Autodesk Inventor part; units mm, degrees
(part 13 of 13)
sketch "Sketch2" plane through (0, 0, 0) normal (0, 1, 0) x (-1, 0, 0)
  line L0 (-22.8128, 17.9045) -> (22.9025, 17.9045)
  line L1 (-26.8635, 14.0674) -> (-26.8635, -13.9573)
  line L2 (-23.0317, -17.859) -> (22.9423, -17.859)
  line L3 (26.7728, 14.0731) -> (26.7728, -14.1827)
  circle A0 centre (-24.1817, 15.2166) radius 1.1494
  circle A1 centre (-24.1817, -15.1773) radius 1.1495
  circle A2 centre (24.091, -15.1773) radius 1.1495
  circle A3 centre (24.091, 15.2166) radius 1.1494
  arc A4 (-22.8128, 17.9045) -> (-26.8635, 14.0674) centre (-22.8128, 13.8478) ccw
  arc A5 (26.7728, 14.0731) -> (22.9025, 17.9045) centre (22.9025, 14.034) ccw
  arc A6 (-26.8635, -13.9573) -> (-23.0317, -17.859) centre (-22.9612, -13.9573) ccw
  arc A7 (22.9423, -17.859) -> (26.7728, -14.1827) centre (23.0934, -14.1827) ccw
  line L4 (-26.8635, 0.055) -> (26.7728, -0.0548) construction
  line L5 (0.0448, 17.9045) -> (-0.0447, -17.859) construction
  line L6 (22.9025, 18.4045) -> (-22.8128, 18.4045)
  arc A8 (-22.8128, 18.4045) -> (-27.3635, 14.0805) centre (-22.8128, 13.8478) ccw
  line L7 (-27.3635, 14.0805) -> (-27.3635, -13.9573)
  arc A9 (-27.3635, -13.9573) -> (-23.0361, -18.359) centre (-22.9612, -13.9573) ccw
  line L8 (-23.0361, -18.359) -> (22.9323, -18.359)
  arc A10 (22.9323, -18.359) -> (27.2728, -14.1827) centre (23.0934, -14.1827) ccw
  line L9 (27.2728, -14.1827) -> (27.2728, 14.0756)
  arc A11 (27.2728, 14.0756) -> (22.9025, 18.4045) centre (22.9025, 14.034) ccw
  line L10 (-22.8128, 20.4045) -> (22.9025, 20.4045)
  arc A12 (29.2728, 14.0842) -> (22.9025, 20.4045) centre (22.9025, 14.034) ccw
  line L11 (29.2728, 14.0842) -> (29.2728, -14.1827)
  arc A13 (22.8975, -20.359) -> (29.2728, -14.1827) centre (23.0934, -14.1827) ccw
  line L12 (22.8975, -20.359) -> (-23.0515, -20.359)
  arc A14 (-29.3635, -13.9573) -> (-23.0515, -20.359) centre (-22.9612, -13.9573) ccw
  line L13 (-29.3635, -13.9573) -> (-29.3635, 14.127)
  arc A15 (-22.8128, 20.4045) -> (-29.3635, 14.127) centre (-22.8128, 13.8478) ccw
  circle A16 centre (-24.1817, 15.2166) radius 1.7494
  arc A17 (-27.3635, 13.2331) -> (-22.2079, 18.4045) centre (-24.1817, 15.2166) ccw
  circle A18 centre (24.091, 15.2166) radius 1.7494
  arc A19 (22.1171, 18.4045) -> (27.2728, 13.2331) centre (24.091, 15.2166) ccw
  circle A20 centre (24.091, -15.1773) radius 1.7495
  arc A21 (27.2728, -13.1938) -> (22.1073, -18.359) centre (24.091, -15.1773) ccw
  circle A22 centre (-24.1817, -15.1773) radius 1.7495
  arc A23 (-22.1981, -18.359) -> (-27.3635, -13.1937) centre (-24.1817, -15.1773) ccw
  arc A24 (-22.2079, 18.4045) -> (-27.3635, 13.2331) centre (-24.1817, 15.2166) ccw
  arc A25 (27.2728, 13.2331) -> (22.1171, 18.4045) centre (24.091, 15.2166) ccw
  arc A26 (22.1073, -18.359) -> (27.2728, -13.1938) centre (24.091, -15.1773) ccw
  arc A27 (-27.3635, -13.1937) -> (-22.1981, -18.359) centre (-24.1817, -15.1773) ccw
  line L14 (15.9339, -12.0278) -> (33.4909, -12.0278)
  line L15 (15.9339, -1.0278) -> (33.4909, -1.0278)
  point P0 (0, 0)
  point P1 (0, 0)
  dimension "d2" = 0.5
  dimension "d3" = 2
  dimension "d4" = 0.6
  dimension "d5" = 2
  dimension "d6" = 0.6
  dimension "d7" = 2
  dimension "d8" = 0.6
  dimension "d9" = 2
  dimension "d10" = 0.6
  dimension "d11" = 2
  dimension "d22" = 2
  dimension "d23" = 11
  constraints: 40 point on circle, 32 end point, 28 centre point, 10 point on line, 8 coincident, 4 midpoint, 4 tangent, 2 horizontal, 2 vertical, 1 parallel, 1 perpendicular, 22 other
  measures "d2" distance between parallel lines of L0 L6
  measures "d3" distance between parallel lines of L6 L10
  measures "d4" radial gap between concentric circles of A0 A16
  measures "d5" radial gap between concentric circles of A16 A17
  measures "d6" radial gap between concentric circles of A3 A18
  measures "d7" radial gap between concentric circles of A18 A19
  measures "d8" radial gap between concentric circles of A2 A20
  measures "d9" radial gap between concentric circles of A20 A21
  measures "d10" radial gap between concentric circles of A1 A22
  measures "d11" radial gap between concentric circles of A22 A23
  measures "d22" distance edge to line of A2 L14
  measures "d23" distance between parallel lines of L14 L15
extrude "Extrusion1" add sketch "Sketch2" along normal blind 1.5 contours A4 L1 A17 L7 A8 L6 L0 | L0 A17 L1 A4 | A17 L6 A19 L0 | L0 A19 L3 L14 A21 L2 A23 L1 A17 | A19 L6 A11 L9 L3 A5 L0 | L0 A5 L3 A19 | L1 A23 L7 A17 | A24 L7 A27 L8 A26 L9 L14 L11 A13 L12 A14 L13 A15 L10 A12 L15 A25 L6 | L6 A8 L7 A24 | A25 L9 A11 L6 | A19 L9 L15 L3 | A23 L2 A6 L1 | L1 A6 L2 A23 L8 A9 L7 | L15 L9 L14 L3 | L2 A21 L8 A23 | L7 A9 L8 A27 | L15 L11 L14 L9 | L14 L9 A21 L3 | L3 A21 L14 | A21 L14 L3 A7 L2 | L2 A7 L3 A21 L9 A10 L8 | L14 A21 | L8 A10 L9 A26 | A0 | A1 | A2 | A3 | A16 | A18 | A20 | A22
extrude "Extrusion2" cut sketch "Sketch2" along normal blind 1.5 contours A0 | A1 | A2 | A3 | A16 | A18 | A20 | A22
extrude "Extrusion3" add sketch "Sketch2" along normal blind 3 contours A4 L1 A17 L7 A8 L6 L0 | L0 A17 L1 A4 | A19 L6 A11 L9 L3 A5 L0 | L0 A5 L3 A19 | L6 A8 L7 A24 | A25 L9 A11 L6 | A23 L2 A6 L1 | L1 A6 L2 A23 L8 A9 L7 | L7 A9 L8 A27 | A21 L14 L3 A7 L2 | L2 A7 L3 A21 L9 A10 L8 | L14 A21 | L8 A10 L9 A26
extrude "Extrusion4" add sketch "Sketch2" along normal blind 5 contours A24 L7 A27 L8 A26 L9 L14 L11 A13 L12 A14 L13 A15 L10 A12 L15 A25 L6 | L6 A8 L7 A24 | A25 L9 A11 L6 | L7 A9 L8 A27 | L15 L11 L14 L9 | L8 A10 L9 A26
ref_plane "Work Plane1" through (0, 1.5, 0) normal (0, 1, 0) x (-1, 0, 0)
sketch "Sketch3" plane through (0, 1.5, 0) normal (0, 1, 0) x (-1, 0, 0)
  line L0 (30.9565, -1.0278) -> (23.8177, -1.0278)
  line L1 (23.8177, -1.0278) -> (23.8177, -12.0278)
  line L2 (23.8177, -12.0278) -> (30.9565, -12.0278)
  line L3 (30.9565, -12.0278) -> (30.9565, -1.0278)
  line L4 (15.9339, -1.0278) -> (33.4909, -1.0278) projected
  line L5 (15.9339, -12.0278) -> (33.4909, -12.0278) projected
  point P0 (0, 0)
  constraints: 8 end point, 2 collinear, 2 parallel, 1 horizontal, 1 perpendicular
extrude "Extrusion5" cut sketch "Sketch3" along normal blind 5
fillet "Fillet1" radius 2 2 edges at (-28.2728, 5, -1.0278) (-28.2728, 5, -12.0278)
sketch "Sketch4" plane through (0, 0, 0) normal (0, -1, 0) x (1, 0, 0)
  line L0 (-22.306, -6.6429) -> (0.6738, -6.6429) construction
  line L1 (0.6738, -6.6429) -> (0.6738, -10.3811) construction
  line L2 (0.6738, -10.3811) -> (-22.306, -10.3811) construction
  line L3 (-22.306, -10.3811) -> (-22.306, -6.6429) construction
  line L4 (-21.9029, 7.8543) -> (-0.5824, 7.8543) construction
  line L5 (-0.5824, 7.8543) -> (-0.5824, 4.3457) construction
  line L6 (-0.5824, 4.3457) -> (-21.9029, 4.3457) construction
  line L7 (-21.9029, 4.3457) -> (-21.9029, 7.8543) construction
  line L8 (-11.3886, -2.1457) -> (-14.0499, -2.1457)
  line L9 (-14.0499, -2.1457) -> (-14.7437, -0.1294)
  line L10 (-14.7437, -0.1294) -> (-18.4417, -0.1294)
  line L11 (-18.4417, -0.1294) -> (-19.1356, -2.1457)
  line L12 (-19.1356, -2.1457) -> (-21.7396, -2.1457)
  line L13 (-21.7396, -2.1457) -> (-18.0499, 7.8543)
  line L14 (-18.0499, 7.8543) -> (-15.0784, 7.8543)
  line L15 (-15.0784, 7.8543) -> (-11.3886, -2.1457)
  line L16 (-15.3641, 1.7073) -> (-16.5968, 5.2828)
  line L17 (-16.5968, 5.2828) -> (-17.8213, 1.7073)
  line L18 (-17.8213, 1.7073) -> (-15.3641, 1.7073)
  spline S0 degree 2 poles (-1.6907, 4.6951) (-1.6907, 4.0257) (-2.1641, 2.7441) (-2.5968, 2.3032) knots 0 0 0 1 2 2 2
  spline S1 degree 2 poles (-2.5968, 2.3032) (-3.1927, 1.7155) (-4.6703, 1.1114) (-5.7641, 1.1114) knots 0 0 0 1 2 2 2
  line L19 (-5.7641, 1.1114) -> (-7.3723, 1.1114)
  line L20 (-7.3723, 1.1114) -> (-7.3723, -2.1457)
  line L21 (-7.3723, -2.1457) -> (-9.9519, -2.1457)
  line L22 (-9.9519, -2.1457) -> (-9.9519, 7.8543)
  line L23 (-9.9519, 7.8543) -> (-5.707, 7.8543)
  spline S2 degree 2 poles (-5.707, 7.8543) (-4.7519, 7.8543) (-3.4376, 7.5277) (-2.9315, 7.193) knots 0 0 0 1 2 2 2
  spline S3 degree 2 poles (-2.9315, 7.193) (-2.3274, 6.8012) (-1.6907, 5.5604) (-1.6907, 4.6951) knots 0 0 0 1 2 2 2
  spline S4 degree 2 poles (-4.3601, 4.6379) (-4.3601, 5.0624) (-4.8172, 5.6665) (-5.1192, 5.789) knots 0 0 0 1 2 2 2
  spline S5 degree 2 poles (-5.1192, 5.789) (-5.5192, 5.9522) (-6.2866, 5.9849) (-6.9315, 5.9849) knots 0 0 0 1 2 2 2
  line L24 (-6.9315, 5.9849) -> (-7.3723, 5.9849)
  line L25 (-7.3723, 5.9849) -> (-7.3723, 2.9971)
  line L26 (-7.3723, 2.9971) -> (-6.6294, 2.9971)
  spline S6 degree 2 poles (-6.6294, 2.9971) (-5.9764, 2.9971) (-5.1192, 3.1604) (-4.8335, 3.3971) knots 0 0 0 1 2 2 2
  spline S7 degree 2 poles (-4.8335, 3.3971) (-4.5805, 3.6175) (-4.3601, 4.2134) (-4.3601, 4.6379) knots 0 0 0 1 2 2 2
  line L27 (10.6195, -2.1457) -> (8.0563, -2.1457)
  line L28 (8.0563, -2.1457) -> (8.0563, 4.5481)
  line L29 (8.0563, 4.5481) -> (6.2032, 0.2053)
  line L30 (6.2032, 0.2053) -> (4.4155, 0.2053)
  line L31 (4.4155, 0.2053) -> (2.5624, 4.5481)
  line L32 (2.5624, 4.5481) -> (2.5624, -2.1457)
  line L33 (2.5624, -2.1457) -> (0.1297, -2.1457)
  line L34 (0.1297, -2.1457) -> (0.1297, 7.8543)
  line L35 (0.1297, 7.8543) -> (3.1257, 7.8543)
  line L36 (3.1257, 7.8543) -> (5.3787, 2.8338)
  line L37 (5.3787, 2.8338) -> (7.6236, 7.8543)
  line L38 (7.6236, 7.8543) -> (10.6195, 7.8543)
  line L39 (10.6195, 7.8543) -> (10.6195, -2.1457)
  spline S8 degree 2 poles (21.7297, 0.9155) (21.7297, 0.189) (21.142, -0.9539) (20.6359, -1.3294) knots 0 0 0 1 2 2 2
  spline S9 degree 2 poles (20.6359, -1.3294) (20.0399, -1.7702) (18.6277, -2.1457) (17.5338, -2.1457) knots 0 0 0 1 2 2 2
  line L40 (17.5338, -2.1457) -> (13.1665, -2.1457)
  line L41 (13.1665, -2.1457) -> (13.1665, 7.8543)
  line L42 (13.1665, 7.8543) -> (17.0522, 7.8543)
  spline S10 degree 2 poles (17.0522, 7.8543) (18.2604, 7.8543) (19.3787, 7.691) (19.9338, 7.4216) knots 0 0 0 1 2 2 2
  spline S11 degree 2 poles (19.9338, 7.4216) (20.5053, 7.1277) (21.0604, 6.1563) (21.0604, 5.5277) knots 0 0 0 1 2 2 2
  spline S12 degree 2 poles (21.0604, 5.5277) (21.0604, 4.8012) (20.293, 3.6992) (19.591, 3.389) knots 0 0 0 1 2 2 2
  line L43 (19.591, 3.389) -> (19.591, 3.3318)
  spline S13 degree 2 poles (19.591, 3.3318) (20.5787, 3.1359) (21.7297, 1.9196) (21.7297, 0.9155) knots 0 0 0 1 2 2 2
  spline S14 degree 2 poles (19.0522, 0.9563) (19.0522, 1.4379) (18.6848, 1.9522) (18.2359, 2.0828) knots 0 0 0 1 2 2 2
  spline S15 degree 2 poles (18.2359, 2.0828) (17.9338, 2.1645) (16.8726, 2.1808) (16.293, 2.1808) knots 0 0 0 1 2 2 2
  line L44 (16.293, 2.1808) -> (15.7297, 2.1808)
  line L45 (15.7297, 2.1808) -> (15.7297, -0.309)
  line L46 (15.7297, -0.309) -> (15.9175, -0.309)
  spline S16 degree 2 poles (15.9175, -0.309) (17.0114, -0.309) (17.9501, -0.2927) (18.342, -0.1294) knots 0 0 0 1 2 2 2
  spline S17 degree 2 poles (18.342, -0.1294) (18.7501, 0.042) (19.0522, 0.5971) (19.0522, 0.9563) knots 0 0 0 1 2 2 2
  spline S18 degree 2 poles (18.4236, 5.0216) (18.4236, 5.2747) (18.1706, 5.7726) (17.8604, 5.8869) knots 0 0 0 1 2 2 2
  spline S19 degree 2 poles (17.8604, 5.8869) (17.5746, 6.0012) (16.7338, 6.0175) (15.9746, 6.0175) knots 0 0 0 1 2 2 2
  line L47 (15.9746, 6.0175) -> (15.7297, 6.0175)
  line L48 (15.7297, 6.0175) -> (15.7297, 3.9032)
  line L49 (15.7297, 3.9032) -> (16.1379, 3.9032)
  spline S20 degree 2 poles (16.1379, 3.9032) (16.7501, 3.9032) (17.6073, 3.9441) (17.8604, 4.0583) knots 0 0 0 1 2 2 2
  spline S21 degree 2 poles (17.8604, 4.0583) (18.2114, 4.2134) (18.4236, 4.7032) (18.4236, 5.0216) knots 0 0 0 1 2 2 2
  line L50 (-17.9435, -10.8225) -> (-19.2007, -10.8225)
  line L51 (-19.2007, -10.8225) -> (-20.2913, -9.3563)
  line L52 (-20.2913, -9.3563) -> (-20.7713, -9.3563)
  line L53 (-20.7713, -9.3563) -> (-20.7713, -10.8225)
  line L54 (-20.7713, -10.8225) -> (-21.7966, -10.8225)
  line L55 (-21.7966, -10.8225) -> (-21.7966, -6.8225)
  line L56 (-21.7966, -6.8225) -> (-20.066, -6.8225)
  spline S22 degree 2 poles (-20.066, -6.8225) (-19.7101, -6.8225) (-19.2007, -6.9041) (-18.9786, -7.038) knots 0 0 0 1 2 2 2
  spline S23 degree 2 poles (-18.9786, -7.038) (-18.7501, -7.1718) (-18.4856, -7.5996) (-18.4856, -7.9229) knots 0 0 0 1 2 2 2
  spline S24 degree 2 poles (-18.4856, -7.9229) (-18.4856, -8.3637) (-18.897, -8.9253) (-19.279, -9.1082) knots 0 0 0 1 2 2 2
  line L57 (-19.279, -9.1082) -> (-17.9435, -10.8225)
  spline S25 degree 2 poles (-19.5533, -8.0469) (-19.5533, -7.8967) (-19.6774, -7.6812) (-19.8276, -7.6192) knots 0 0 0 1 2 2 2
  spline S26 degree 2 poles (-19.8276, -7.6192) (-19.9321, -7.5767) (-20.2129, -7.5571) (-20.399, -7.5571) knots 0 0 0 1 2 2 2
  line L58 (-20.399, -7.5571) -> (-20.7713, -7.5571)
  line L59 (-20.7713, -7.5571) -> (-20.7713, -8.6347)
  line L60 (-20.7713, -8.6347) -> (-20.4546, -8.6347)
  spline S27 degree 2 poles (-20.4546, -8.6347) (-20.2064, -8.6347) (-19.8733, -8.5857) (-19.759, -8.5008) knots 0 0 0 1 2 2 2
  spline S28 degree 2 poles (-19.759, -8.5008) (-19.6513, -8.4159) (-19.5533, -8.2167) (-19.5533, -8.0469) knots 0 0 0 1 2 2 2
  spline S29 degree 2 poles (-14.4595, -9.3139) (-14.4595, -10.0584) (-15.328, -10.9171) (-16.1117, -10.9171) knots 0 0 0 1 2 2 2
  spline S30 degree 2 poles (-16.1117, -10.9171) (-16.8986, -10.9171) (-17.7672, -10.0584) (-17.7672, -9.3139) knots 0 0 0 1 2 2 2
  spline S31 degree 2 poles (-17.7672, -9.3139) (-17.7672, -8.5661) (-16.8921, -7.7106) (-16.1117, -7.7106) knots 0 0 0 1 2 2 2
  spline S32 degree 2 poles (-16.1117, -7.7106) (-15.3215, -7.7106) (-14.4595, -8.5694) (-14.4595, -9.3139) knots 0 0 0 1 2 2 2
  spline S33 degree 2 poles (-15.6513, -10.0486) (-15.5566, -9.931) (-15.4619, -9.6078) (-15.4619, -9.3204) knots 0 0 0 1 2 2 2
  spline S34 degree 2 poles (-15.4619, -9.3204) (-15.4619, -9.0559) (-15.5599, -8.6967) (-15.6448, -8.589) knots 0 0 0 1 2 2 2
  spline S35 degree 2 poles (-15.6448, -8.589) (-15.7297, -8.478) (-15.9746, -8.3865) (-16.1117, -8.3865) knots 0 0 0 1 2 2 2
  spline S36 degree 2 poles (-16.1117, -8.3865) (-16.2521, -8.3865) (-16.4709, -8.4616) (-16.5721, -8.5759) knots 0 0 0 1 2 2 2
  spline S37 degree 2 poles (-16.5721, -8.5759) (-16.6603, -8.6804) (-16.7648, -9.0429) (-16.7648, -9.3204) knots 0 0 0 1 2 2 2
  spline S38 degree 2 poles (-16.7648, -9.3204) (-16.7648, -9.5686) (-16.6733, -9.931) (-16.5852, -10.0388) knots 0 0 0 1 2 2 2
  spline S39 degree 2 poles (-16.5852, -10.0388) (-16.497, -10.1433) (-16.2586, -10.2412) (-16.1052, -10.2412) knots 0 0 0 1 2 2 2
  spline S40 degree 2 poles (-16.1052, -10.2412) (-15.9746, -10.2412) (-15.7329, -10.1531) (-15.6513, -10.0486) knots 0 0 0 1 2 2 2
  spline S41 degree 2 poles (-10.6195, -9.2714) (-10.6195, -9.9833) (-11.4064, -10.8812) (-11.9941, -10.8812) knots 0 0 0 1 2 2 2
  spline S42 degree 2 poles (-11.9941, -10.8812) (-12.2456, -10.8812) (-12.6244, -10.7735) (-12.7974, -10.6723) knots 0 0 0 1 2 2 2
  line L61 (-12.7974, -10.6723) -> (-12.8366, -10.8225)
  line L62 (-12.8366, -10.8225) -> (-13.7672, -10.8225)
  line L63 (-13.7672, -10.8225) -> (-13.7672, -6.6429)
  line L64 (-13.7672, -6.6429) -> (-12.7974, -6.6429)
  line L65 (-12.7974, -6.6429) -> (-12.7974, -8.122)
  spline S43 degree 2 poles (-12.7974, -8.122) (-12.5754, -7.9425) (-12.1117, -7.7237) (-11.808, -7.7237) knots 0 0 0 1 2 2 2
  spline S44 degree 2 poles (-11.808, -7.7237) (-11.2366, -7.7237) (-10.6195, -8.5465) (-10.6195, -9.2714) knots 0 0 0 1 2 2 2
  spline S45 degree 2 poles (-11.6154, -9.2943) (-11.6154, -8.8927) (-11.8897, -8.4584) (-12.239, -8.4584) knots 0 0 0 1 2 2 2
  spline S46 degree 2 poles (-12.239, -8.4584) (-12.3762, -8.4584) (-12.6668, -8.54) (-12.7974, -8.6184) knots 0 0 0 1 2 2 2
  line L66 (-12.7974, -8.6184) -> (-12.7974, -10.1269)
  spline S47 degree 2 poles (-12.7974, -10.1269) (-12.6929, -10.1661) (-12.5068, -10.1923) (-12.3729, -10.1923) knots 0 0 0 1 2 2 2
  spline S48 degree 2 poles (-12.3729, -10.1923) (-11.9909, -10.1923) (-11.6154, -9.7416) (-11.6154, -9.2943) knots 0 0 0 1 2 2 2
  spline S49 degree 2 poles (-6.835, -9.3139) (-6.835, -10.0584) (-7.7035, -10.9171) (-8.4872, -10.9171) knots 0 0 0 1 2 2 2
  spline S50 degree 2 poles (-8.4872, -10.9171) (-9.2741, -10.9171) (-10.1427, -10.0584) (-10.1427, -9.3139) knots 0 0 0 1 2 2 2
  spline S51 degree 2 poles (-10.1427, -9.3139) (-10.1427, -8.5661) (-9.2676, -7.7106) (-8.4872, -7.7106) knots 0 0 0 1 2 2 2
  spline S52 degree 2 poles (-8.4872, -7.7106) (-7.697, -7.7106) (-6.835, -8.5694) (-6.835, -9.3139) knots 0 0 0 1 2 2 2
  spline S53 degree 2 poles (-8.0268, -10.0486) (-7.9321, -9.931) (-7.8374, -9.6078) (-7.8374, -9.3204) knots 0 0 0 1 2 2 2
  spline S54 degree 2 poles (-7.8374, -9.3204) (-7.8374, -9.0559) (-7.9354, -8.6967) (-8.0203, -8.589) knots 0 0 0 1 2 2 2
  spline S55 degree 2 poles (-8.0203, -8.589) (-8.1052, -8.478) (-8.3501, -8.3865) (-8.4872, -8.3865) knots 0 0 0 1 2 2 2
  spline S56 degree 2 poles (-8.4872, -8.3865) (-8.6276, -8.3865) (-8.8464, -8.4616) (-8.9476, -8.5759) knots 0 0 0 1 2 2 2
  spline S57 degree 2 poles (-8.9476, -8.5759) (-9.0358, -8.6804) (-9.1403, -9.0429) (-9.1403, -9.3204) knots 0 0 0 1 2 2 2
  spline S58 degree 2 poles (-9.1403, -9.3204) (-9.1403, -9.5686) (-9.0488, -9.931) (-8.9607, -10.0388) knots 0 0 0 1 2 2 2
  spline S59 degree 2 poles (-8.9607, -10.0388) (-8.8725, -10.1433) (-8.6341, -10.2412) (-8.4807, -10.2412) knots 0 0 0 1 2 2 2
  spline S60 degree 2 poles (-8.4807, -10.2412) (-8.3501, -10.2412) (-8.1084, -10.1531) (-8.0268, -10.0486) knots 0 0 0 1 2 2 2
  spline S61 degree 2 poles (-2.6652, -9.598) (-2.6652, -9.8886) (-2.9003, -10.3457) (-3.1027, -10.4959) knots 0 0 0 1 2 2 2
  spline S62 degree 2 poles (-3.1027, -10.4959) (-3.3411, -10.6723) (-3.906, -10.8225) (-4.3435, -10.8225) knots 0 0 0 1 2 2 2
  line L67 (-4.3435, -10.8225) -> (-6.0905, -10.8225)
  line L68 (-6.0905, -10.8225) -> (-6.0905, -6.8225)
  line L69 (-6.0905, -6.8225) -> (-4.5362, -6.8225)
  spline S63 degree 2 poles (-4.5362, -6.8225) (-4.0529, -6.8225) (-3.6056, -6.8878) (-3.3835, -6.9955) knots 0 0 0 1 2 2 2
  spline S64 degree 2 poles (-3.3835, -6.9955) (-3.155, -7.1131) (-2.9329, -7.5016) (-2.9329, -7.7531) knots 0 0 0 1 2 2 2
  spline S65 degree 2 poles (-2.9329, -7.7531) (-2.9329, -8.0437) (-3.2399, -8.4845) (-3.5207, -8.6086) knots 0 0 0 1 2 2 2
  line L70 (-3.5207, -8.6086) -> (-3.5207, -8.6314)
  spline S66 degree 2 poles (-3.5207, -8.6314) (-3.1256, -8.7098) (-2.6652, -9.1963) (-2.6652, -9.598) knots 0 0 0 1 2 2 2
  spline S67 degree 2 poles (-3.7362, -9.5816) (-3.7362, -9.389) (-3.8831, -9.1833) (-4.0627, -9.131) knots 0 0 0 1 2 2 2
  spline S68 degree 2 poles (-4.0627, -9.131) (-4.1835, -9.0984) (-4.608, -9.0918) (-4.8399, -9.0918) knots 0 0 0 1 2 2 2
  line L71 (-4.8399, -9.0918) -> (-5.0652, -9.0918)
  line L72 (-5.0652, -9.0918) -> (-5.0652, -10.0878)
  line L73 (-5.0652, -10.0878) -> (-4.9901, -10.0878)
  spline S69 degree 2 poles (-4.9901, -10.0878) (-4.5525, -10.0878) (-4.177, -10.0812) (-4.0203, -10.0159) knots 0 0 0 1 2 2 2
  spline S70 degree 2 poles (-4.0203, -10.0159) (-3.857, -9.9474) (-3.7362, -9.7253) (-3.7362, -9.5816) knots 0 0 0 1 2 2 2
  spline S71 degree 2 poles (-3.9876, -7.9555) (-3.9876, -7.8543) (-4.0888, -7.6551) (-4.2129, -7.6094) knots 0 0 0 1 2 2 2
  spline S72 degree 2 poles (-4.2129, -7.6094) (-4.3272, -7.5637) (-4.6635, -7.5571) (-4.9672, -7.5571) knots 0 0 0 1 2 2 2
  line L74 (-4.9672, -7.5571) -> (-5.0652, -7.5571)
  line L75 (-5.0652, -7.5571) -> (-5.0652, -8.4029)
  line L76 (-5.0652, -8.4029) -> (-4.9019, -8.4029)
  spline S73 degree 2 poles (-4.9019, -8.4029) (-4.657, -8.4029) (-4.3141, -8.3865) (-4.2129, -8.3408) knots 0 0 0 1 2 2 2
  spline S74 degree 2 poles (-4.2129, -8.3408) (-4.0725, -8.2788) (-3.9876, -8.0829) (-3.9876, -7.9555) knots 0 0 0 1 2 2 2
  line L77 (0.2377, -8.7261) -> (0.1528, -8.7261)
  spline S75 degree 2 poles (0.1528, -8.7261) (0.0907, -8.7033) (-0.1835, -8.6837) (-0.275, -8.6837) knots 0 0 0 1 2 2 2
  spline S76 degree 2 poles (-0.275, -8.6837) (-0.4807, -8.6837) (-0.7974, -8.7359) (-0.9803, -8.8012) knots 0 0 0 1 2 2 2
  line L78 (-0.9803, -8.8012) -> (-0.9803, -10.8225)
  line L79 (-0.9803, -10.8225) -> (-1.9501, -10.8225)
  line L80 (-1.9501, -10.8225) -> (-1.9501, -7.8053)
  line L81 (-1.9501, -7.8053) -> (-0.9803, -7.8053)
  line L82 (-0.9803, -7.8053) -> (-0.9803, -8.2494)
  spline S77 degree 2 poles (-0.9803, -8.2494) (-0.6603, -7.9751) (-0.1901, -7.7955) (0.0091, -7.7955) knots 0 0 0 1 2 2 2
  spline S78 degree 2 poles (0.0091, -7.7955) (0.0614, -7.7955) (0.1887, -7.802) (0.2377, -7.8053) knots 0 0 0 1 2 2 2
  line L83 (0.2377, -7.8053) -> (0.2377, -8.7261)
  line L84 (2.974, -8.7261) -> (2.8891, -8.7261)
  spline S79 degree 2 poles (2.8891, -8.7261) (2.8271, -8.7033) (2.5528, -8.6837) (2.4614, -8.6837) knots 0 0 0 1 2 2 2
  spline S80 degree 2 poles (2.4614, -8.6837) (2.2556, -8.6837) (1.9389, -8.7359) (1.7561, -8.8012) knots 0 0 0 1 2 2 2
  line L85 (1.7561, -8.8012) -> (1.7561, -10.8225)
  line L86 (1.7561, -10.8225) -> (0.7863, -10.8225)
  line L87 (0.7863, -10.8225) -> (0.7863, -7.8053)
  line L88 (0.7863, -7.8053) -> (1.7561, -7.8053)
  line L89 (1.7561, -7.8053) -> (1.7561, -8.2494)
  spline S81 degree 2 poles (1.7561, -8.2494) (2.0761, -7.9751) (2.5463, -7.7955) (2.7454, -7.7955) knots 0 0 0 1 2 2 2
  spline S82 degree 2 poles (2.7454, -7.7955) (2.7977, -7.7955) (2.925, -7.802) (2.974, -7.8053) knots 0 0 0 1 2 2 2
  line L90 (2.974, -7.8053) -> (2.974, -8.7261)
  line L91 (6.4548, -10.8225) -> (5.485, -10.8225)
  line L92 (5.485, -10.8225) -> (5.485, -10.509)
  spline S83 degree 2 poles (5.485, -10.509) (5.2369, -10.7114) (4.8026, -10.9074) (4.5152, -10.9074) knots 0 0 0 1 2 2 2
  spline S84 degree 2 poles (4.5152, -10.9074) (3.9667, -10.9074) (3.3071, -10.0584) (3.3071, -9.3367) knots 0 0 0 1 2 2 2
  spline S85 degree 2 poles (3.3071, -9.3367) (3.3071, -8.9547) (3.5291, -8.3604) (3.7218, -8.1482) knots 0 0 0 1 2 2 2
  spline S86 degree 2 poles (3.7218, -8.1482) (3.9046, -7.9457) (4.4271, -7.7237) (4.685, -7.7237) knots 0 0 0 1 2 2 2
  spline S87 degree 2 poles (4.685, -7.7237) (4.9561, -7.7237) (5.3022, -7.838) (5.485, -7.9294) knots 0 0 0 1 2 2 2
  line L93 (5.485, -7.9294) -> (5.485, -6.6429)
  line L94 (5.485, -6.6429) -> (6.4548, -6.6429)
  line L95 (6.4548, -6.6429) -> (6.4548, -10.8225)
  line L96 (5.485, -9.9931) -> (5.485, -8.5106)
  spline S88 degree 2 poles (5.485, -8.5106) (5.3838, -8.4682) (5.1585, -8.429) (5.0638, -8.429) knots 0 0 0 1 2 2 2
  spline S89 degree 2 poles (5.0638, -8.429) (4.685, -8.429) (4.303, -8.9057) (4.303, -9.3269) knots 0 0 0 1 2 2 2
  spline S90 degree 2 poles (4.303, -9.3269) (4.303, -9.771) (4.6099, -10.1727) (4.9463, -10.1727) knots 0 0 0 1 2 2 2
  spline S91 degree 2 poles (4.9463, -10.1727) (5.0769, -10.1727) (5.374, -10.0747) (5.485, -9.9931) knots 0 0 0 1 2 2 2
  line L97 (8.4107, -10.8225) -> (7.405, -10.8225)
  line L98 (7.405, -10.8225) -> (7.405, -9.7678)
  line L99 (7.405, -9.7678) -> (8.4107, -9.7678)
  line L100 (8.4107, -9.7678) -> (8.4107, -10.8225)
  spline S92 degree 2 poles (10.9283, -10.9041) (10.5332, -10.9041) (9.8801, -10.7147) (9.6385, -10.5188) knots 0 0 0 1 2 2 2
  spline S93 degree 2 poles (9.6385, -10.5188) (9.4001, -10.3229) (9.1356, -9.7286) (9.1356, -9.3269) knots 0 0 0 1 2 2 2
  spline S94 degree 2 poles (9.1356, -9.3269) (9.1356, -8.9057) (9.4165, -8.2918) (9.6712, -8.0927) knots 0 0 0 1 2 2 2
  spline S95 degree 2 poles (9.6712, -8.0927) (9.9161, -7.9) (10.5528, -7.7237) (10.8989, -7.7237) knots 0 0 0 1 2 2 2
  spline S96 degree 2 poles (10.8989, -7.7237) (11.2059, -7.7237) (11.7283, -7.8576) (11.9536, -7.9653) knots 0 0 0 1 2 2 2
  line L101 (11.9536, -7.9653) -> (11.9536, -8.7914)
  line L102 (11.9536, -8.7914) -> (11.8165, -8.7914)
  spline S97 degree 2 poles (11.8165, -8.7914) (11.761, -8.7425) (11.601, -8.6118) (11.4867, -8.5498) knots 0 0 0 1 2 2 2
  spline S98 degree 2 poles (11.4867, -8.5498) (11.3756, -8.491) (11.1144, -8.4127) (10.9414, -8.4127) knots 0 0 0 1 2 2 2
  spline S99 degree 2 poles (10.9414, -8.4127) (10.5528, -8.4127) (10.1381, -8.9057) (10.1381, -9.3269) knots 0 0 0 1 2 2 2
  spline S100 degree 2 poles (10.1381, -9.3269) (10.1381, -9.7645) (10.5659, -10.2151) (10.9544, -10.2151) knots 0 0 0 1 2 2 2
  spline S101 degree 2 poles (10.9544, -10.2151) (11.1373, -10.2151) (11.4312, -10.1302) (11.5259, -10.0747) knots 0 0 0 1 2 2 2
  spline S102 degree 2 poles (11.5259, -10.0747) (11.6173, -10.0225) (11.7577, -9.9016) (11.8165, -9.8461) knots 0 0 0 1 2 2 2
  line L103 (11.8165, -9.8461) -> (11.9536, -9.8461)
  line L104 (11.9536, -9.8461) -> (11.9536, -10.669)
  spline S103 degree 2 poles (11.9536, -10.669) (11.725, -10.7767) (11.2287, -10.9041) (10.9283, -10.9041) knots 0 0 0 1 2 2 2
  spline S104 degree 2 poles (15.6793, -9.3139) (15.6793, -10.0584) (14.8107, -10.9171) (14.0271, -10.9171) knots 0 0 0 1 2 2 2
  spline S105 degree 2 poles (14.0271, -10.9171) (13.2401, -10.9171) (12.3716, -10.0584) (12.3716, -9.3139) knots 0 0 0 1 2 2 2
  spline S106 degree 2 poles (12.3716, -9.3139) (12.3716, -8.5661) (13.2467, -7.7106) (14.0271, -7.7106) knots 0 0 0 1 2 2 2
  spline S107 degree 2 poles (14.0271, -7.7106) (14.8173, -7.7106) (15.6793, -8.5694) (15.6793, -9.3139) knots 0 0 0 1 2 2 2
  spline S108 degree 2 poles (14.4875, -10.0486) (14.5822, -9.931) (14.6769, -9.6078) (14.6769, -9.3204) knots 0 0 0 1 2 2 2
  spline S109 degree 2 poles (14.6769, -9.3204) (14.6769, -9.0559) (14.5789, -8.6967) (14.494, -8.589) knots 0 0 0 1 2 2 2
  spline S110 degree 2 poles (14.494, -8.589) (14.4091, -8.478) (14.1642, -8.3865) (14.0271, -8.3865) knots 0 0 0 1 2 2 2
  spline S111 degree 2 poles (14.0271, -8.3865) (13.8867, -8.3865) (13.6679, -8.4616) (13.5667, -8.5759) knots 0 0 0 1 2 2 2
  spline S112 degree 2 poles (13.5667, -8.5759) (13.4785, -8.6804) (13.374, -9.0429) (13.374, -9.3204) knots 0 0 0 1 2 2 2
  spline S113 degree 2 poles (13.374, -9.3204) (13.374, -9.5686) (13.4654, -9.931) (13.5536, -10.0388) knots 0 0 0 1 2 2 2
  spline S114 degree 2 poles (13.5536, -10.0388) (13.6418, -10.1433) (13.8801, -10.2412) (14.0336, -10.2412) knots 0 0 0 1 2 2 2
  spline S115 degree 2 poles (14.0336, -10.2412) (14.1642, -10.2412) (14.4059, -10.1531) (14.4875, -10.0486) knots 0 0 0 1 2 2 2
  line L105 (19.3169, -8.6837) -> (19.3169, -10.8225)
  line L106 (19.3169, -10.8225) -> (18.3471, -10.8225)
  line L107 (18.3471, -10.8225) -> (18.3471, -9.3139)
  spline S116 degree 2 poles (18.3471, -9.3139) (18.3471, -9.0951) (18.3242, -8.7849) (18.2785, -8.6902) knots 0 0 0 1 2 2 2
  spline S117 degree 2 poles (18.2785, -8.6902) (18.2295, -8.5923) (18.0336, -8.5041) (17.8573, -8.5041) knots 0 0 0 1 2 2 2
  spline S118 degree 2 poles (17.8573, -8.5041) (17.7136, -8.5041) (17.4459, -8.6184) (17.3381, -8.6837) knots 0 0 0 1 2 2 2
  line L108 (17.3381, -8.6837) -> (17.3381, -10.8225)
  line L109 (17.3381, -10.8225) -> (16.3683, -10.8225)
  line L110 (16.3683, -10.8225) -> (16.3683, -7.8053)
  line L111 (16.3683, -7.8053) -> (17.3381, -7.8053)
  line L112 (17.3381, -7.8053) -> (17.3381, -8.1384)
  spline S119 degree 2 poles (17.3381, -8.1384) (17.5863, -7.9425) (18.0434, -7.7237) (18.321, -7.7237) knots 0 0 0 1 2 2 2
  spline S120 degree 2 poles (18.321, -7.7237) (18.6181, -7.7237) (19.072, -7.9882) (19.2026, -8.2461) knots 0 0 0 1 2 2 2
  spline S121 degree 2 poles (19.2026, -8.2461) (19.4899, -8.0045) (20.0385, -7.7237) (20.2997, -7.7237) knots 0 0 0 1 2 2 2
  spline S122 degree 2 poles (20.2997, -7.7237) (20.7895, -7.7237) (21.2956, -8.3082) (21.2956, -8.86) knots 0 0 0 1 2 2 2
  line L113 (21.2956, -8.86) -> (21.2956, -10.8225)
  line L114 (21.2956, -10.8225) -> (20.3259, -10.8225)
  line L115 (20.3259, -10.8225) -> (20.3259, -9.3139)
  spline S123 degree 2 poles (20.3259, -9.3139) (20.3259, -9.0918) (20.3063, -8.7849) (20.2573, -8.6902) knots 0 0 0 1 2 2 2
  spline S124 degree 2 poles (20.2573, -8.6902) (20.2116, -8.5923) (20.0156, -8.5041) (19.8361, -8.5041) knots 0 0 0 1 2 2 2
  spline S125 degree 2 poles (19.8361, -8.5041) (19.7152, -8.5041) (19.4834, -8.5857) (19.3169, -8.6837) knots 0 0 0 1 2 2 2
  point P0 (0, 0)
  constraints: 4 other
emboss "Emboss2" sketch "Sketch4" operation cut depth 0.54 direction (0, 1, 0)
body "Solid1"
